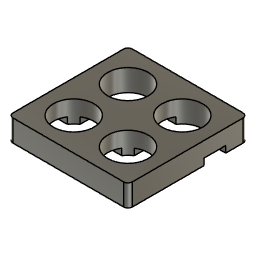
EE-SPRO3_Battery_holder v1 (Autodesk Fusion 360 design; units mm, degrees)
Autodesk Fusion 360 part; units mm, degrees
sketch "Sketch1" plane through (0, 0, 0) normal (0, 0, 1) x (1, 0, 0)
  circle A0 centre (0, 0) radius 9.35
  circle A1 centre (25, 0) radius 9.35
  circle A2 centre (0, 25) radius 9.35
  circle A3 centre (25, 25) radius 9.35
  line L0 (-15, -15) -> (40, -15)
  line L1 (40, -15) -> (40, 40)
  line L2 (40, 40) -> (-15, 40)
  line L3 (-15, 40) -> (-15, -15)
  dimension "d1" = 18.7
  dimension "d4" = 25
  dimension "d5" = 25
  constraint coincident A0.centre origin
  constraint horizontal L0
  constraint vertical L1
  constraint horizontal L2
  constraint vertical L3
  measures "d1" diameter of A0
extrude "Extrude1" add sketch "Sketch1" along normal blind 10
fillet "Fillet1" radius 2 4 edges at (-15, -15, 5) (-15, 40, 5) (40, -15, 5) (40, 40, 5)
sketch "Sketch2" plane through (0, 0, 0) normal (0, 0, -1) x (1, 0, 0)
  circle A0 centre (25, 0) radius 9.35
  circle A1 centre (0, 0) radius 9.35
  circle A2 centre (25, -25) radius 9.35
  circle A3 centre (0, -25) radius 9.35
  arc A4 (38, -40) -> (40, -38) centre (38, -38) ccw
  line L0 (40, -38) -> (40, 13)
  arc A5 (40, 13) -> (38, 15) centre (38, 13) ccw
  line L1 (38, 15) -> (-13, 15)
  arc A6 (-13, 15) -> (-15, 13) centre (-13, 13) ccw
  line L2 (-15, 13) -> (-15, -38)
  arc A7 (-15, -38) -> (-13, -40) centre (-13, -38) ccw
  line L3 (-13, -40) -> (38, -40)
  line L4 (-5, -5) -> (5, -5)
  line L5 (5, -5) -> (5, -20)
  line L6 (5, -20) -> (-5, -20)
  line L7 (-5, -20) -> (-5, -5)
  line L8 (5, -5) -> (20, -5)
  line L9 (20, -5) -> (20, 5)
  line L10 (20, 5) -> (5, 5)
  line L11 (5, 5) -> (5, -5)
  line L12 (20, -5) -> (30, -5)
  line L13 (30, -5) -> (30, -20)
  line L14 (30, -20) -> (20, -20)
  line L15 (20, -20) -> (20, -5)
  line L16 (5, -20) -> (20, -20)
  line L17 (20, -20) -> (20, -30)
  line L18 (20, -30) -> (5, -30)
  line L19 (5, -30) -> (5, -20)
  line L20 (-20, 5) -> (-5, 5)
  line L21 (-5, 5) -> (-5, -5)
  line L22 (-5, -5) -> (-20, -5)
  line L23 (-20, -5) -> (-20, 5)
  line L24 (30, -20) -> (45, -20)
  line L25 (45, -20) -> (45, -30)
  line L26 (45, -30) -> (30, -30)
  line L27 (30, -30) -> (30, -20)
  constraint horizontal L4
  constraint vertical L5
  constraint horizontal L6
  constraint vertical L7
  constraint horizontal L8
  constraint vertical L9
  constraint horizontal L10
  constraint vertical L11
  constraint horizontal L12
  constraint vertical L13
  constraint horizontal L14
  constraint vertical L15
  constraint horizontal L16
  constraint vertical L17
  constraint horizontal L18
  constraint vertical L19
  constraint horizontal L20
  constraint vertical L21
  constraint horizontal L22
  constraint vertical L23
  constraint horizontal L24
  constraint vertical L25
  constraint horizontal L26
  constraint vertical L27
extrude "Extrude2" cut sketch "Sketch2" against normal blind 3 contours A0 A1 L8 L10 | A0 A2 L13 L15 | A1 L2 L20 L22 | A2 L0 L24 L26 | A1 A3 L5 L7 | A2 A3 L16 L18
